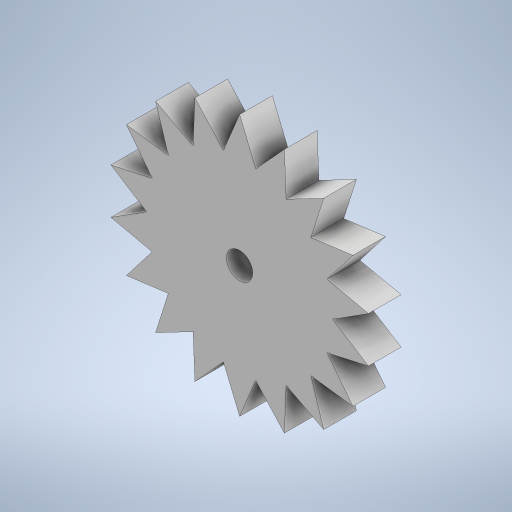
# Autodesk Inventor part: Drive Gear
Saved by Autodesk Inventor 2023 (Build 270158030, 158C)
## iProperties
Created: 2022-09-22
Part Number: Drive Gear
Material: Generic
Document SubType Name: Modeling
Designer: cjj5381
Density: 1 g/cm^3
Appearance: Default
Author: cjj5381
Autodesk Inventor part; units mm, degrees
ref_plane "YZ Plane" through (0, 0, 0) normal (1, 0, 0) x (0, 1, 0)
ref_plane "XZ Plane" through (0, 0, 0) normal (0, 1, 0) x (-1, 0, 0)
ref_plane "XY Plane" through (0, 0, 0) normal (0, 0, 1) x (1, 0, 0)
sketch "Sketch2" plane through (0, 0, 0) normal (0, 0, 1) x (1, 0, 0)
  circle A0 centre (0, 0) radius 10
  dimension "d0" = 20
  constraints: 1 centre point, 1 coincident
  measures "d0" diameter of A0
extrude "Extrusion1" add sketch "Sketch2" along normal blind 5
sketch "Sketch3" plane through (0, 0, 5) normal (0, 0, 1) x (1, 0, 0)
  line L0 (0, 0) -> (0, 9.5351)
  line L1 (0, 20) -> (-4.6081, 8.875)
  circle A0 centre (0, 0) radius 10 projected
  line L2 (0, 20) -> (4.6081, 8.875)
  arc A1 (4.6081, 8.875) -> (-4.6081, 8.875) centre (0, 0) ccw
  point P0 (0, 10)
  dimension "d3" = 45
  dimension "d4" = 10
  constraints: 6 end point, 5 point on circle, 1 centre point, 1 concentric, 1 point on line, 1 symmetric about line, 1 vertical
  measures "d3" angle of L2 L1
  measures "d4" distance of point (0, 10) L1.start
extrude "Extrusion2" add sketch "Sketch3" against normal up to surface (5 mm away) contours L2 A0 L1
pattern_circular "Circular Pattern1" count 18 over 360 about axis through (0, 0, 0) along (0, 0, 1) of "Extrusion2"
sketch "Sketch4" plane through (0, 0, 0) normal (0, 0, -1) x (-1, 0, 0)
  point P0 (0, 0)
  point P1 (0, 0)
  constraints: 1 coincident
hole "Hole1" at (0, 0, 0) at (0, 0, 0) direction (0, 0, 1) diameter 4 end through all
body "Solid1"
